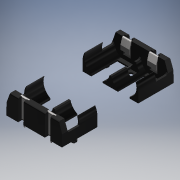
# Autodesk Inventor part: PSU test long
Saved by Autodesk Inventor 2017 (Build 210142000, 142)
## iProperties
Part Number: PSU test long
Material: Acetalharz, schwarz
Document SubType Name: Modeling
Designer: David
Density: 1.425 g/cm^3
Appearance: Glatt - schwarz
Author: David
Autodesk Inventor part; units mm, degrees
sketch "Skizze1" plane through (0, 0, 0) normal (0, 1, 0) x (-1, 0, 0)
  line L0 (17.5181, 7.4549) -> (-17.5181, 7.4549)
  line L1 (19.8882, 0.5715) -> (19.8882, -7.4549)
  line L2 (19.8882, -7.4549) -> (-19.8882, -7.4549)
  line L3 (-19.8882, -7.4549) -> (-19.8882, 0.5715)
  line L4 (-19.8882, 0.5715) -> (-17.5181, 7.4549)
  line L5 (17.5181, 7.4549) -> (19.8882, 0.5715)
  line L6 (-19.8882, -7.4549) -> (-19.8882, 7.4549) construction
  line L7 (-19.8882, 7.4549) -> (19.8882, 7.4549) construction
  line L8 (19.8882, 7.4549) -> (19.8882, -7.4549) construction
  line L9 (-19.8882, 7.4549) -> (19.8882, -7.4549) construction
  point P0 (0, 0)
  point P1 (0, 0)
  point P2 (0, 0)
  constraints: 20 end point, 1 coincident, 1 horizontal, 1 midpoint, 1 parallel, 1 vertical, 1 other
extrude "Extrusion1" add sketch "Skizze1" along normal mid plane 79.966
sketch "Skizze6" plane through (19.8882, -39.983, -7.4549) normal (1, 0, 0) x (0, 0, -1)
  arc A0 (-14.9098, 1.2587) -> (-13.9115, 0.2428) centre (-13.8938, 1.2587) ccw
  line L0 (-14.9098, 1.2587) -> (-14.9098, 4.0855) construction
  spline S0 degree 3 poles (-8.6868, 4.0855) (-8.488, 4.0855) (-8.2765, 4.1255) (-7.8884, 4.2868) (-7.7116, 4.4081) (-7.4331, 4.6873) (-7.3123, 4.8637) (-7.1517, 5.2511) (-7.112, 5.4621) (-7.112, 5.6603) knots 0 0 0 0 0.250545 0.250545 0.50109 0.50109 0.750545 0.750545 1 1 1 1
  line L1 (-8.6868, 4.0855) -> (-14.9098, 4.0855)
  line L2 (0, 0) -> (0, 79.966)
  line L3 (-18.1411, 39.983) -> (3.0235, 39.983) construction
  line L4 (-7.112, 5.6603) -> (-7.112, 39.983)
  line L5 (-14.9098, 4.0855) -> (-14.9098, 39.983)
  line L6 (-14.9098, 0) -> (-14.9098, 79.966)
  line L7 (-14.9098, 39.983) -> (-7.112, 39.983)
  line L8 (0, 0) -> (-8.0264, 0)
  line L9 (-14.9098, 0) -> (0, 0)
  line L10 (0, 0) -> (-13.9115, 0.2428)
  line L11 (-14.9098, 1.2587) -> (-14.9098, 0)
  point P0 (-7.4549, 39.983)
  constraints: 16 end point, 2 collinear, 2 horizontal, 2 point on circle, 1 centre point, 1 midpoint, 1 point on line, 1 vertical, 4 other
extrude "Extrusion5" cut sketch "Skizze6" against normal through all
sketch "Skizze7" plane through (-19.6608, -35.8975, 1.2319) normal (0, 1, 0) x (1, 0, 0)
  arc A0 (5.9702, 7.7022) -> (0.9651, 0) centre (10.0977, -0.4572) ccw
  line L0 (19.2303, 0) -> (20.0913, 0)
  arc A1 (19.2303, 0) -> (14.2252, 7.7022) centre (10.0977, -0.4572) ccw
  line L1 (5.9702, 7.6962) -> (14.2252, 7.6962)
  line L2 (0, 0) -> (0.9651, 0)
  line L3 (0, 0) -> (2.1428, -6.223)
  arc A2 (25.0964, 7.7022) -> (20.0913, 0) centre (29.2239, -0.4572) ccw
  line L4 (25.0964, 7.6962) -> (33.3514, 7.6962)
  line L5 (2.1428, -6.223) -> (37.1789, -6.223)
  line L6 (37.1789, -6.223) -> (39.3216, 0)
  line L7 (38.3565, 0) -> (39.3216, 0)
  arc A3 (38.3565, 0) -> (33.3514, 7.7022) centre (29.2239, -0.4572) ccw
  line L8 (25.0964, 7.6962) -> (25.0964, 7.7022)
  line L9 (33.3514, 7.6962) -> (33.3514, 7.7022)
  line L10 (14.2252, 7.6962) -> (14.2252, 7.7022)
  line L11 (5.9702, 7.7022) -> (5.9702, 7.6962)
  point P0 (19.6608, 1.2319)
  point P1 (37.1789, -6.223)
  point P2 (19.6608, 1.2319)
  point P3 (19.5729, -2.4475)
  point P4 (37.1789, -6.223)
  constraints: 24 end point, 8 point on circle, 4 centre point, 2 parallel
extrude "Extrusion6" cut sketch "Skizze7" along normal up to surface (35.8975 mm away)
sketch "Skizze8" plane through (-17.5181, -38.7243, 7.4549) normal (0, 0, 1) x (1, 0, 0)
  line L0 (14.3431, 6.4718) -> (14.3431, 12.8218)
  line L1 (16.8703, 6.4718) -> (14.3431, 6.4718)
  line L2 (18.1658, 6.4718) -> (16.8703, 6.4718)
  line L3 (20.6931, 6.4718) -> (18.1658, 6.4718)
  line L4 (20.6931, 12.8218) -> (20.6931, 6.4718)
  line L5 (18.1658, 12.8218) -> (20.6931, 12.8218)
  line L6 (16.8703, 12.8218) -> (18.1658, 12.8218)
  line L7 (14.3431, 12.8218) -> (16.8703, 12.8218)
  circle A0 centre (17.5181, 9.6468) radius 1.5875
  line L8 (6.05, -1.2587) -> (6.05, 1.6331)
  line L9 (6.05, 1.6331) -> (9.86, 1.6331)
  line L10 (9.86, 1.6331) -> (9.86, -1.2587)
  line L11 (28.9862, 1.6331) -> (28.9862, -1.2587)
  line L12 (25.1762, 1.6331) -> (28.9862, 1.6331)
  line L13 (25.1762, -1.2587) -> (25.1762, 1.6331)
  line L14 (22.9537, 5.5409) -> (31.2087, 5.5409)
  line L15 (22.9537, 5.5409) -> (22.9537, 38.7243)
  line L16 (31.2087, 5.5409) -> (31.2087, 38.7243)
  line L17 (3.8275, 5.5409) -> (12.0825, 5.5409)
  line L18 (3.8275, 5.5409) -> (3.8275, 38.7243)
  line L19 (12.0825, 5.5409) -> (12.0825, 38.7243)
  line L20 (4.653, 1.2521) -> (6.05, 1.2521)
  line L21 (4.653, 2.8269) -> (4.653, 1.2521)
  line L22 (9.86, 1.2521) -> (11.257, 1.2521)
  line L23 (11.257, 1.2521) -> (11.257, 2.8269)
  line L24 (23.7792, 1.2521) -> (25.1762, 1.2521)
  line L25 (23.7792, 2.8269) -> (23.7792, 1.2521)
  line L26 (24.2872, 2.8269) -> (23.7792, 2.8269)
  line L27 (24.2872, 2.8269) -> (24.2872, 1.6331)
  line L28 (23.7792, 1.6331) -> (24.2872, 1.6331)
  line L29 (30.3832, 2.8269) -> (29.8752, 2.8269)
  line L30 (29.8752, 1.6331) -> (29.8752, 2.8269)
  line L31 (29.8752, 1.6331) -> (30.3832, 1.6331)
  line L32 (30.3832, 1.2521) -> (30.3832, 2.8269)
  line L33 (28.9862, 1.2521) -> (30.3832, 1.2521)
  line L34 (10.749, 1.6331) -> (11.257, 1.6331)
  line L35 (10.749, 2.8269) -> (10.749, 1.6331)
  line L36 (11.257, 2.8269) -> (10.749, 2.8269)
  line L37 (4.653, 1.6331) -> (5.161, 1.6331)
  line L38 (5.161, 1.6331) -> (5.161, 2.8269)
  line L39 (5.161, 2.8269) -> (4.653, 2.8269)
  line L40 (10.749, 2.8269) -> (5.161, 2.8269)
  line L41 (29.8752, 2.8269) -> (24.2872, 2.8269)
  line L42 (17.9486, 2.8269) -> (22.9537, 2.8269) projected
  line L43 (25.1762, 1.6331) -> (24.2872, 1.6331)
  line L44 (29.8752, 1.6331) -> (28.9862, 1.6331)
  line L45 (35.0361, 2.8269) -> (0, 2.8269) projected
  line L46 (10.749, 1.6331) -> (9.86, 1.6331)
  line L47 (6.05, 1.6331) -> (5.161, 1.6331)
  line L48 (0, 38.7243) -> (35.0361, 38.7243) projected
  line L49 (3.8275, 38.7243) -> (12.0825, 38.7243)
  line L50 (22.9537, 38.7243) -> (31.2087, 38.7243)
  line L51 (6.05, -1.2587) -> (9.86, -1.2587)
  line L52 (35.3798, -1.0158) -> (-0.3437, -1.0158) projected
  line L53 (28.9862, -1.2587) -> (25.1762, -1.2587)
  line L54 (-2.3701, -1.2587) -> (37.4063, -1.2587) projected
  point P0 (17.5181, 38.7243)
  point P1 (17.606, 39.6773)
  constraints: 100 end point, 4 collinear, 4 point on line, 2 parallel, 1 centre point, 1 horizontal
extrude "Extrusion7" cut sketch "Skizze8" against normal blind 11.1 contours L47 L38 L40 L35 L46 L9 | L43 L27 L41 L30 L44 L12
extrude "Extrusion8" cut sketch "Skizze8" against normal blind 3.175 contours L37 L21 L39 L38 | L35 L36 L23 L34 | L28 L25 L26 L27 | L30 L29 L32 L31
extrude "Extrusion9" cut sketch "Skizze8" against normal blind 14.072 contours L20 L21 L37 L47 L8 | L46 L34 L23 L22 L10 | L24 L25 L28 L43 L13 | L11 L44 L31 L32 L33
extrude "Extrusion10" cut sketch "Skizze8" against normal through all contours A0 | L8 L9 L10 L52 | L52 L10 L51 L8 | L52 L11 L53 L13 | L13 L12 L11 L52 | L15 L48 L16 L14 | L18 L48 L19 L17
extrude "Extrusion11" cut sketch "Skizze8" against normal blind 13.925 contours L0 L7 L6 L5 L4 L3 L2 L1
ref_plane "Arbeitsebene4" through (5.4356, -27.3125, -6.4643) normal (0, 1, 0) x (1, 0, 0)
sketch "Skizze9" plane through (5.4356, -27.3125, -6.4643) normal (0, 1, 0) x (1, 0, 0)
  arc A0 (-25.3238, -6.1214) -> (-23.7614, -11.5824) centre (-14.9987, -6.1214) ccw
  arc A1 (-23.9141, -6.1214) -> (-23.5067, -11.5041) centre (-14.9987, -8.1534) ccw
  line L0 (-23.7614, -11.5824) -> (-23.5067, -11.5041)
  arc A2 (12.6355, -11.5041) -> (13.0429, -6.1214) centre (4.1275, -8.1534) ccw
  arc A3 (12.8902, -11.5824) -> (14.4526, -6.1214) centre (4.1275, -6.1214) ccw
  line L1 (12.8902, -11.5824) -> (12.6355, -11.5041)
  line L2 (14.4526, -6.1214) -> (13.0429, -6.1214)
  line L3 (-23.9141, -6.1214) -> (-25.3238, -6.1214)
  point P0 (-5.4356, -6.4643)
  point P1 (-5.5235, -10.1437)
  point P2 (14.4526, 0.9906)
  point P3 (14.4526, 0.9906)
  constraints: 8 end point, 8 point on circle, 4 centre point, 1 collinear, 1 horizontal
extrude "Extrusion12" add sketch "Skizze9" along normal blind 12.7
ref_plane "Arbeitsebene5" through (9.5631, -38.7243, 7.4549) normal (1, 0, 0) x (0, 0, -1)
sketch "Skizze10" plane through (9.5631, -38.7243, 7.4549) normal (1, 0, 0) x (0, 0, -1)
  line L0 (7.874, 3.9097) -> (7.874, 4.2145)
  line L1 (4.9784, 4.2145) -> (7.874, 4.2145)
  line L2 (4.9784, 3.9097) -> (7.874, 3.9097)
  arc A0 (4.9784, 3.9097) -> (4.8014, 3.8845) centre (4.9784, 3.2747) ccw
  arc A1 (4.9784, 4.2145) -> (4.7164, 4.1772) centre (4.9784, 3.2747) ccw
  line L3 (0.7176, 3.0165) -> (4.7164, 4.1772)
  line L4 (0.8624, 2.7411) -> (4.8014, 3.8845)
  arc A2 (0.8624, 2.7411) -> (1.1684, 1.5569) centre (1.1211, 2.1763) ccw
  arc A3 (0.7176, 3.0165) -> (1.1684, 1.2521) centre (1.1684, 2.1919) ccw
  line L5 (6.5786, 1.5569) -> (1.1684, 1.5569)
  line L6 (6.5786, 1.2521) -> (1.1684, 1.2521)
  line L7 (6.5786, 1.2521) -> (8.1534, 1.2521)
  line L8 (6.5786, 1.5569) -> (14.0716, 1.5569)
  line L9 (14.072, 1.5569) -> (15.342, 1.5552)
  spline S0 degree 3 poles (17.628, 1.5552) (17.2656, 1.4042) (16.8773, 1.3266) (16.0927, 1.3266) (15.7044, 1.4042) (15.342, 1.5552) knots 0 0 0 0 0.5 0.5 1 1 1 1 construction
  spline S1 degree 3 poles (15.342, 1.5552) (15.7044, 1.7062) (16.0927, 1.7838) (16.8773, 1.7838) (17.2656, 1.7062) (17.628, 1.5552) knots 0 0 0 0 0.5 0.5 1 1 1 1 construction
  line L10 (17.628, 1.5552) -> (17.9074, 1.5552)
  line L11 (18.3896, 1.5552) -> (17.9074, 1.5552)
  line L12 (18.3896, 1.2504) -> (17.907, 1.2504)
  spline S2 degree 3 poles (15.342, 1.5552) (15.7044, 1.7062) (16.0927, 1.7838) (16.8773, 1.7838) (17.2656, 1.7062) (17.628, 1.5552) knots 0 0 0 0 0.5 0.5 1 1 1 1 construction
  spline S3 degree 3 poles (15.3416, 1.2504) (15.704, 1.4014) (16.0923, 1.479) (16.8769, 1.479) (17.2652, 1.4014) (17.6276, 1.2504) knots 0 0 0 0 0.5 0.5 1 1 1 1 construction
  spline S4 degree 3 poles (17.6276, 1.2504) (17.2652, 1.0994) (16.8769, 1.0218) (16.0923, 1.0218) (15.704, 1.0994) (15.3416, 1.2504) knots 0 0 0 0 0.5 0.5 1 1 1 1 construction
  line L13 (17.907, 1.2504) -> (17.6276, 1.2504)
  line L14 (15.3416, 1.2504) -> (17.6276, 1.2504)
  line L15 (17.628, 1.5552) -> (15.342, 1.5552)
  line L16 (18.3896, 1.5552) -> (18.3896, 1.2504)
  line L17 (14.072, 1.5569) -> (14.072, 1.2521)
  line L18 (14.072, 1.2521) -> (15.3416, 1.2504)
  line L19 (14.072, 1.5569) -> (14.0716, 1.5569)
  line L20 (11.1, 2.8269) -> (3.175, 2.8269)
  line L21 (0, 1.2521) -> (14.072, 1.2521)
  line L22 (8.1534, 1.2521) -> (14.072, 1.2521)
  line L23 (6.191, 4.2145) -> (9.0866, 4.2145)
  line L24 (7.874, 4.2145) -> (8.3078, 3.8741)
  point P0 (7.4549, 38.7243)
  point P1 (14.9098, -1.2587)
  point P2 (14.9098, -1.2587)
  dimension "d55" = 0.2688
  constraints: 46 end point, 8 point on circle, 5 horizontal alignment, 4 centre point, 3 parallel, 3 tangent, 1 coincident, 1 collinear, 1 horizontal, 1 perpendicular, 1 point on line, 18 other
mirror "Spiegeln4" about plane through (0, 0, 0) normal (0, 1, 0) of "Extrusion5", "Extrusion6", "Extrusion7", "Extrusion8", "Extrusion9", "Extrusion10", "Extrusion11", "Extrusion12"
extrude "Extrusion14" add sketch "Skizze10" along normal mid plane 6.35 contours L2 A0 L4 A2 L5 L8 L17 L21 L7 L6 A3 L3 A1 L1 L0
extrude "Extrusion15" add sketch "Skizze10" along normal mid plane 0.965 contours L9 L15 L10 L11 L16 L12 L13 L14 L18 L17
pattern_linear "Rechteckige Anordnung1" count 2 spacing 19.126 along (-1, 0, 0) of "Extrusion14", "Extrusion15"
mirror "Spiegeln5" about plane through (0, 0, 0) normal (0, 1, 0) of "Extrusion14", "Extrusion15", "Rechteckige Anordnung1"
ref_plane "Arbeitsebene6" through (17.5002, -39.8429, 0.5715) normal (1, 0, 0) x (0, 0, -1)
sketch "Skizze12" plane through (17.5002, -39.8429, 0.5715) normal (1, 0, 0) x (0, 0, -1)
  line L0 (8.0264, -0.1401) -> (8.0264, 79.8259) construction
  arc A0 (8.7884, 9.3048) -> (8.0264, 8.5428) centre (8.7884, 8.5428) ccw
  line L1 (9.8044, 9.3048) -> (8.7884, 9.3048)
  line L2 (9.8044, 9.3048) -> (9.8044, 8.9238)
  line L3 (10.0076, 8.9238) -> (9.8044, 8.9238)
  arc A1 (10.0076, 8.9238) -> (11.4554, 10.2385) centre (10.1346, 10.2385) ccw
  line L4 (8.0264, 12.3528) -> (8.0264, 9.1778) construction
  line L5 (8.0264, 8.5428) -> (8.0264, 10.7653)
  line L6 (8.0264, 73.0264) -> (8.0264, 6.6594) construction
  line L7 (11.4554, 10.7653) -> (8.0264, 10.7653)
  line L8 (11.4554, 10.7653) -> (11.4554, 10.2385)
  point P0 (0.5715, 39.8429)
  constraints: 12 end point, 4 point on circle, 2 centre point, 2 vertical, 1 collinear, 1 horizontal, 1 midpoint, 1 point on line, 1 tangent
revolve "Umdrehung2" add sketch "Skizze12" angle 360 about axis through (17.5002, -29.0776, -10.8839) along (0, 0, 1)
ref_plane "Arbeitsebene7" through (7.6581, -39.983, -8.7389) normal (0, 0, -1) x (-1, 0, 0)
sketch "Skizze15" plane through (7.6581, -39.983, -8.7389) normal (0, 0, -1) x (-1, 0, 0)
  line L0 (-11.3665, 10.499) -> (-11.3665, 9.8609)
  line L1 (-10.1777, 10.499) -> (-11.3665, 10.499)
  line L2 (-10.1777, 10.499) -> (-9.5073, 10.499)
  line L3 (-8.3185, 10.499) -> (-9.5073, 10.499)
  line L4 (-8.3185, 9.6376) -> (-8.3185, 10.499)
  line L5 (-8.3185, 11.3118) -> (-8.3185, 12.0782)
  line L6 (-9.5073, 11.3118) -> (-8.3185, 11.3118)
  line L7 (-9.5073, 11.3118) -> (-10.1777, 11.3118)
  line L8 (-11.3665, 11.3118) -> (-10.1777, 11.3118)
  line L9 (-11.3665, 11.95) -> (-11.3665, 11.3118)
  arc A0 (-11.3665, 11.95) -> (-11.3665, 9.8609) centre (-9.8459, 10.9054) ccw
  arc A1 (-8.3185, 9.6376) -> (-8.3185, 12.0782) centre (-9.7105, 10.8579) ccw
  circle A2 centre (-9.8421, 10.9054) radius 1.8415 projected
  circle A3 centre (-9.8421, 10.9054) radius 1.8415 projected
  circle A4 centre (-9.8421, 10.9054) radius 0.5268 projected
  circle A5 centre (-9.8421, 10.9054) radius 1.8415 projected
  point P0 (7.6581, 39.983)
  point P1 (-12.2301, 0)
  point P2 (-8.3185, 11.9391)
  point P3 (-11.3665, 11.9391)
  point P4 (-12.2301, 0)
  constraints: 20 end point, 4 point on circle, 2 centre point, 1 collinear, 2 other
extrude "Extrusion17" cut sketch "Skizze15" along normal through all contours L0 A2 L9 L8 A4 L1 | L0 A0 L9 A2 | A4 L7 L2 | A2 L5 A1 L4 | L4 L3 A4 L6 L5 A2
pattern_circular "Runde Anordnung1" count 2 over 360 about axis through (0, 0, -10) along (0, 0, 1) of "Extrusion17", "Umdrehung2"
sketch "Skizze16" plane through (7.6581, -39.983, -7.4549) normal (0, 0, -1) x (-1, 0, 0)
  circle A0 centre (25.1587, 2.6631) radius 0.7874
  point P0 (7.6581, 39.983)
  point P1 (27.5463, 0)
  point P2 (27.5463, 0)
  constraints: 1 centre point
ref_plane "Arbeitsebene8" through (-17.5006, -37.3199, -7.4549) normal (-1, 0, 0) x (0, 0, 1)
sketch "Skizze17" plane through (-17.5006, -37.3199, -7.4549) normal (-1, 0, 0) x (0, 0, 1)
  line L0 (-0.7874, -0.7874) -> (0, -0.7874)
  line L1 (0, 0) -> (0, -0.7874)
  line L2 (0, 0) -> (-1.5748, 0)
  arc A0 (-1.5748, 0) -> (-0.7874, -0.7874) centre (-0.7874, 0) ccw
  point P0 (7.4549, 37.3199)
  point P1 (0, -2.6631)
  point P2 (0, -2.6631)
  constraints: 6 end point, 2 point on circle, 1 centre point, 1 perpendicular
revolve "Umdrehung3" add sketch "Skizze17" angle 360 about axis through (-17.5006, -37.3199, -7.4549) along (0, 0, -1)
sketch "Skizze11" plane through (-19.8882, 14.6125, -0.3429) normal (0, -1, 0) x (1, 0, 0)
  line L0 (-3.3384, 8.3463) -> (40.4232, 8.3463)
  line L1 (40.4232, 8.3463) -> (40.4232, -8.1309)
  line L2 (40.4232, -8.1309) -> (-3.3384, -8.1309)
  line L3 (-3.3384, -8.1309) -> (-3.3384, 8.3463)
  point P0 (19.8882, 0.3429)
  constraints: 8 end point, 2 parallel, 1 horizontal, 1 perpendicular
extrude "Extrusion16" cut sketch "Skizze11" along normal up to surface (29.2249 mm away)
